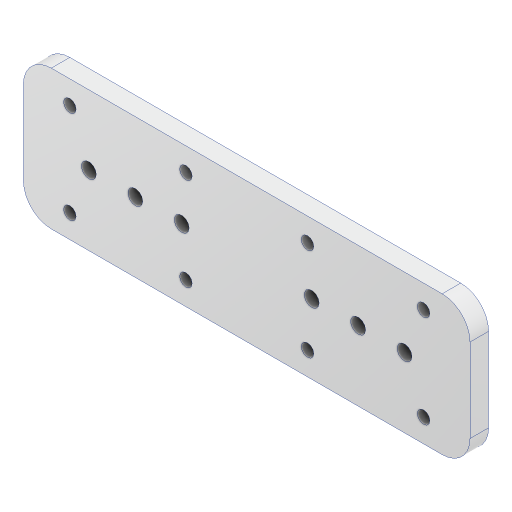
# Autodesk Inventor part: lm가이드가이드
Saved by Autodesk Inventor 2023.2 (Build 272271000, 271)
## iProperties
Created: 2022-12-30
Part Number: lm가이드가이드
Material: 알루미늄 6061
Document SubType Name: Modeling
Designer: BAEK
Density: 2.7 g/cm^3
Appearance: 알루미늄 - 평지
Author: BAEK
Autodesk Inventor part; units mm, degrees
ref_plane "YZ Plane" through (0, 0, 0) normal (1, 0, 0) x (0, 1, 0)
ref_plane "XZ Plane" through (0, 0, 0) normal (0, 1, 0) x (-1, 0, 0)
ref_plane "XY Plane" through (0, 0, 0) normal (0, 0, 1) x (1, 0, 0)
sketch "스케치1" plane through (0, 0, 0) normal (0, 0, 1) x (1, 0, 0)
  line L0 (-48.1, 15) -> (48.1, 15)
  line L1 (48.1, 15) -> (48.1, -15)
  line L2 (48.1, -15) -> (-48.1, -15)
  line L3 (-48.1, -15) -> (-48.1, 15)
  line L4 (-48.1, 15) -> (48.1, -15) construction
  line L5 (48.1, 15) -> (-48.1, -15) construction
  point P0 (0, 0)
  dimension "d0" = 96.2
  dimension "d1" = 30
  constraints: 12 end point, 2 midpoint, 2 parallel, 1 horizontal, 1 perpendicular
  measures "d0" distance of L1.end L2.end
  measures "d1" distance of L0.end L1.end
extrude "돌출1" add sketch "스케치1" along normal blind 4
sketch "스케치2" plane through (0, 0, 4) normal (0, 0, 1) x (1, 0, 0)
  line L0 (-48.1, 15) -> (-48.1, -15) projected
  line L1 (-48.1, 0) -> (48.1, 0) construction
  line L2 (48.1, -15) -> (48.1, 15) projected
  circle A0 centre (-24, 0) radius 1.6
  circle A1 centre (-34, 0) radius 1.6
  circle A2 centre (14, 0) radius 1.6
  circle A3 centre (24, 0) radius 1.6
  circle A4 centre (34, 0) radius 1.6
  circle A5 centre (-14, 0) radius 1.6
  point P0 (0, 0)
  point P1 (0, 0)
  dimension "d5" = 3.2
  dimension "d6" = 3.2
  dimension "d7" = 3.2
  dimension "d8" = 3.2
  dimension "d9" = 14
  dimension "d10" = 10
  dimension "d11" = 3.2
  dimension "d12" = 3.2
  dimension "d13" = 10
  dimension "d14" = 14
  dimension "d15" = 10
  dimension "d16" = 10
  constraints: 6 centre point, 2 midpoint, 10 other
  measures "d5" diameter of A0
  measures "d6" diameter of A1
  measures "d7" diameter of A2
  measures "d8" diameter of A3
  measures "d9" distance of A2.centre point (0, 0)
  measures "d10" distance of A3.centre A2.centre
  measures "d11" diameter of A4
  measures "d12" diameter of A5
  measures "d13" distance of A4.centre A3.centre
  measures "d14" distance of A5.centre point (0, 0)
  measures "d15" distance of A0.centre A5.centre
  measures "d16" distance of A1.centre A0.centre
extrude "돌출2" cut sketch "스케치2" against normal blind 4
fillet "모깎기1" radius 6 4 edges at (-48.1, 15, 2) (-48.1, -15, 2) (48.1, -15, 2) (48.1, 15, 2)
sketch "스케치3" plane through (0, 0, 4) normal (0, 0, 1) x (1, 0, 0)
  arc A0 (48.1, 9) -> (42.1, 15) centre (42.1, 9) ccw projected
  line L0 (42.1, 15) -> (-42.1, 15) projected
  arc A1 (-42.1, 15) -> (-48.1, 9) centre (-42.1, 9) ccw projected
  line L1 (-48.1, 9) -> (-48.1, -9) projected
  arc A2 (-48.1, -9) -> (-42.1, -15) centre (-42.1, -9) ccw projected
  line L2 (-42.1, -15) -> (42.1, -15) projected
  arc A3 (42.1, -15) -> (48.1, -9) centre (42.1, -9) ccw projected
  line L3 (48.1, -9) -> (48.1, 9) projected
  circle A4 centre (-14, 0) radius 1.6 projected
  circle A5 centre (34, 0) radius 1.6 projected
  circle A6 centre (-24, 0) radius 1.6 projected
  circle A7 centre (14, 0) radius 1.6 projected
  circle A8 centre (24, 0) radius 1.6 projected
  circle A9 centre (-34, 0) radius 1.6 projected
  circle A10 centre (-38.1, 10) radius 1.35
  circle A11 centre (-13.1, 10) radius 1.35
  circle A12 centre (-38.1, -10) radius 1.35
  circle A13 centre (-13.1, -10) radius 1.35
  line L4 (0, 0) -> (0, 15)
  line L5 (42.1, 15) -> (-42.1, 15) projected
  line L6 (48.1, 9) -> (48.1, -9)
  circle A14 centre (38.1, 10) radius 1.35
  circle A15 centre (13.1, 10) radius 1.35
  circle A16 centre (38.1, -10) radius 1.35
  circle A17 centre (13.1, -10) radius 1.35
  dimension "d20" = 2.7
  dimension "d21" = 2.7
  dimension "d22" = 2.7
  dimension "d23" = 2.7
  dimension "d24" = 25
  dimension "d25" = 25
  dimension "d26" = 20
  dimension "d27" = 10
  dimension "d28" = 10
  constraints: 8 centre point, 4 end point, 4 symmetric about line, 2 horizontal alignment, 1 midpoint, 1 vertical alignment, 4 other
  measures "d20" diameter of A10
  measures "d21" diameter of A11
  measures "d22" diameter of A12
  measures "d23" diameter of A13
  measures "d24" distance of A10.centre A11.centre
  measures "d25" distance of A13.centre A12.centre
  measures "d26" distance of A10.centre A12.centre
  measures "d27" vertical distance of A9.centre A10.centre
  measures "d28" distance from line of L1 A10.centre
extrude "돌출3" cut sketch "스케치3" against normal blind 4 contours A10 | A11 | A12 | A13 | A14 | A15 | A16 | A17
